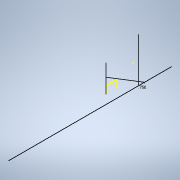
# Autodesk Inventor part: backRamp
Saved by Autodesk Inventor 2021 (Build 250183000, 183)
## iProperties
Created: 2020-09-18
Part Number: backRamp
Material: Generic
Document SubType Name: Modeling
Designer: deli
Density: 1 g/cm^3
Appearance: Default
Author: deli
Autodesk Inventor part; units mm, degrees
ref_plane "YZ Plane" through (0, 0, 0) normal (1, 0, 0) x (0, 1, 0)
ref_plane "XZ Plane" through (0, 0, 0) normal (0, 1, 0) x (-1, 0, 0)
ref_plane "XY Plane" through (0, 0, 0) normal (0, 0, 1) x (1, 0, 0)
sketch "Sketch1" plane through (0, 0, 0) normal (1, 0, 0) x (0, 1, 0)
  line L0 (-18.2699, 90.9518) -> (-43.6699, 90.9518) projected
  line L1 (-43.6699, 90.9518) -> (-43.6699, 87.7768) projected
  line L2 (-43.6699, 87.7768) -> (-21.4449, 87.7768) projected
  line L3 (-21.4449, 87.7768) -> (-21.4449, 56.0268) projected
  line L4 (-21.4449, 56.0268) -> (-43.6699, 56.0268) projected
  line L5 (-43.6699, 56.0268) -> (-43.6699, 52.8518) projected
  line L6 (-43.6699, 52.8518) -> (-18.2699, 52.8518) projected
  line L7 (-18.2699, 52.8518) -> (-18.2699, 90.9518) projected
  line L8 (-73.6331, -37.3594) -> (5.1124, 90.9518)
  line L9 (-73.6331, 413.8255) -> (-73.6331, -18.3094)
  line L10 (-73.6331, -18.3094) -> (-73.6331, -127.5459)
  line L11 (-43.6699, 90.9518) -> (46.9661, 90.9518)
  line L12 (-73.6331, -18.3094) -> (73.7672, -18.3094)
  line L13 (-73.6331, -18.3094) -> (-52.9491, 217.9518)
  line L14 (-52.9491, 217.9518) -> (-56.112, 218.2287)
  line L15 (-56.112, 218.2287) -> (-73.6331, 18.0955)
  point P0 (0, 0)
  dimension "d0" = 19.05
  dimension "d1" = 20.32
  dimension "d2" = 0
  dimension "d3" = 3.175
  dimension "d6" = 127
  constraints: 16 end point, 5 point on line, 2 horizontal, 2 vertical, 1 parallel, 1 perpendicular, 3 other
  measures "d0" distance from line of L8.start L12
  measures "d1" distance from line of L13 L0.end
  measures "d2" distance from line of L13.start L12
  measures "d3" distance of L13.end L14.end
  measures "d6" distance from line of L11 L13.end
extrude "Extrusion1" add sketch "Sketch1" along normal mid plane 256.0066 contours L9 L15 L14 L13
body "Solid1"
